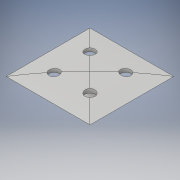
# Autodesk Inventor part: thumper-bumper-trigger
Saved by Autodesk Inventor 2017 (Build 210142000, 142)
## iProperties
Created: 2017-02-22
Part Number: thumper-bumper-trigger
Material: Generic
Document SubType Name: Modeling
Designer: John
Density: 1 g/cm^3
Appearance: Default
Author: John
Autodesk Inventor part; units mm, degrees
ref_plane "YZ Plane" through (0, 0, 0) normal (1, 0, 0) x (0, 1, 0)
ref_plane "XZ Plane" through (0, 0, 0) normal (0, 1, 0) x (-1, 0, 0)
ref_plane "XY Plane" through (0, 0, 0) normal (0, 0, 1) x (1, 0, 0)
sketch "Sketch1" plane through (0, 0, 0) normal (0, 1, 0) x (-1, 0, 0)
  line L0 (37.5, -37.5) -> (-37.5, -37.5)
  line L1 (-37.5, -37.5) -> (-37.5, 37.5)
  line L2 (-37.5, 37.5) -> (37.5, 37.5)
  line L3 (37.5, 37.5) -> (37.5, -37.5)
  line L4 (37.5, -37.5) -> (-37.5, 37.5) construction
  line L5 (-37.5, -37.5) -> (37.5, 37.5) construction
  point P0 (0, 0)
  dimension "d0" = 75
  dimension "d1" = 75
  constraints: 12 end point, 2 midpoint, 2 parallel, 1 horizontal, 1 perpendicular
  measures "d0" distance of L1.end L2.end
  measures "d1" distance of L0.end L1.end
sketch "Sketch2" plane through (0, 0, 0) normal (0, 1, 0) x (-1, 0, 0)
  line L0 (-25, -25) -> (25, -25)
  line L1 (25, -25) -> (25, 25)
  line L2 (25, 25) -> (-25, 25)
  line L3 (-25, 25) -> (-25, -25)
  line L4 (-25, -25) -> (25, 25) construction
  line L5 (25, -25) -> (-25, 25) construction
  point P0 (0, 0)
  dimension "d2" = 50
  dimension "d3" = 50
  constraints: 12 end point, 2 midpoint, 2 parallel, 1 horizontal, 1 perpendicular
  measures "d2" distance of L2.end L1.end
  measures "d3" distance of L1.end L0.end
extrude "Extrusion1" add sketch "Sketch1" along normal blind 4
extrude "Extrusion2" [suppressed]
sketch "Sketch3" plane through (37.5, 0, 37.5) normal (1, 0, 0) x (0, 0, -1)
  line L0 (75, 4) -> (0, 4) projected
  line L1 (0, 0) -> (75, 0) projected
  line L2 (0, 0) -> (75, 0)
  arc A0 (75, 0) -> (0, 0) centre (37.5, -173.7812) ccw
  point P0 (37.5, 4)
  constraints: 3 point on circle, 2 end point, 1 centre point, 1 horizontal, 1 midpoint
extrude "Extrusion3" cut sketch "Sketch3" against normal through all keep common part
sketch "Sketch4" plane through (37.5, 0, -37.5) normal (0, 0, -1) x (-1, 0, 0)
  line L0 (75, 0) -> (75, 4) projected
  line L1 (0, 0) -> (75, 0)
  line L2 (0, 0) -> (0, 4) projected
  line L3 (75, 0) -> (0, 0) projected
  arc A0 (75, 0) -> (0, 0) centre (37.5, -173.7813) ccw
  point P0 (37.5, 0)
  constraints: 2 end point, 2 point on circle, 1 centre point, 1 horizontal
extrude "Extrusion4" cut sketch "Sketch4" against normal through all keep common part
sketch "Sketch5" plane through (0, 0, 0) normal (0, -1, 0) x (1, 0, 0)
  circle A0 centre (0, 0) radius 4.5
  dimension "d14" = 9
  constraints: 1 centre point, 1 coincident
  measures "d14" diameter of A0
extrude "Extrusion5" add sketch "Sketch5" along normal blind 25
sketch "Sketch6" plane through (0, 0, 0) normal (0, -1, 0) x (1, 0, 0)
  circle A0 centre (-16, -16) radius 4.5
  circle A1 centre (16, 16) radius 4.5
  line L0 (0, 0) -> (37.5, 37.5) projected
  circle A2 centre (16, -16) radius 4.5
  circle A3 centre (-16, 16) radius 4.5
  point P0 (0, 0)
  dimension "d17" = 9
  dimension "d18" = 9
  dimension "d19" = 16
  dimension "d20" = 16
  dimension "d21" = 16
  dimension "d22" = 16
  dimension "d25" = 9
  dimension "d26" = 9
  constraints: 4 centre point, 1 coincident
  measures "d17" diameter of A0
  measures "d18" diameter of A1
  measures "d19" horizontal distance of point (0, 0) A0.centre
  measures "d20" horizontal distance of A1.centre point (0, 0)
  measures "d21" horizontal distance of point (0, 0) A1.centre
  measures "d22" horizontal distance of point (0, 0) A0.centre
  measures "d25" diameter of A2
  measures "d26" diameter of A3
extrude "Extrusion6" cut sketch "Sketch6" against normal through all
body "Solid1"
